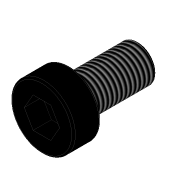
# Autodesk Inventor part: M3 x 8 Socket Head Bolt
Saved by Autodesk Inventor 2020 (Build 240168000, 168)
## iProperties
Created: 2021-07-20
Part Number: M3 x 8 Socket Head Bolt
Material: Generic
Document SubType Name: Modeling
Designer: Coy
Density: 1 g/cm^3
Appearance: Anodized - Black
Author: Coy
Autodesk Inventor part; units mm, degrees
ref_plane "YZ Plane" through (0, 0, 0) normal (1, 0, 0) x (0, 1, 0)
ref_plane "XZ Plane" through (0, 0, 0) normal (0, 1, 0) x (-1, 0, 0)
ref_plane "XY Plane" through (0, 0, 0) normal (0, 0, 1) x (1, 0, 0)
sketch "Sketch1" plane through (0, 0, 0) normal (0, 0, 1) x (1, 0, 0)
  circle A0 centre (0, 0) radius 3.45
  line L0 (0.9671, 1.675) -> (1.9341, 0)
  line L1 (1.9341, 0) -> (0.9671, -1.675)
  line L2 (0.9671, -1.675) -> (-0.9671, -1.675)
  line L3 (-0.9671, -1.675) -> (-1.9341, 0)
  line L4 (-1.9341, 0) -> (-0.9671, 1.675)
  line L5 (-0.9671, 1.675) -> (0.9671, 1.675)
  dimension "d0" = 6.9
  dimension "d1" = 3.35
  constraints: 12 end point, 2 coincident, 1 centre point, 13 other
  measures "d0" diameter of A0
  measures "d1" distance between parallel lines of L2 L5
extrude "Extrusion1" add sketch "Sketch1" against normal blind 2
sketch "Sketch2" plane through (0, 0, -2) normal (0, 0, -1) x (-1, 0, 0)
  circle A0 centre (0, 0) radius 3.45 projected
extrude "Extrusion2" add sketch "Sketch2" along normal blind 1
sketch "Sketch3" plane through (0, 0, -3) normal (0, 0, -1) x (-1, 0, 0)
  circle A0 centre (0, 0) radius 2
  dimension "d6" = 4
  constraints: 1 centre point, 1 coincident
  measures "d6" diameter of A0
extrude "Extrusion3" add sketch "Sketch3" along normal blind 7.5
fillet "Fillet1" radius 0.2 3 edges at (3.45, 0, -3) (-3.45, 0, 0) (2, 0, -10.5)
thread "Thread1" size "M3x0.5" class "6g" standard "ANSI Metric M Profile" full length
body "Solid1"
